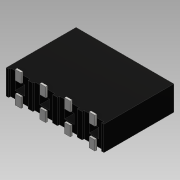
# Autodesk Inventor part: fciconnect-91601-304
Saved by Autodesk Inventor 2016 (Build 200138000, 138)
## iProperties
Created: 2016-06-08
Part Number: fciconnect-91601-304
Material: Generic
Document SubType Name: Modeling
Designer: admin
Density: 1 g/cm^3
Appearance: Default
Mass: 0.150532 g
Surface Area: 3.43025 cm^2
Volume: 0.150532 cm^3
Author: admin
Autodesk Inventor part; units mm, degrees
ref_plane "YZ Plane" through (0, 0, 0) normal (1, 0, 0) x (0, 1, 0)
ref_plane "XZ Plane" through (0, 0, 0) normal (0, 1, 0) x (-1, 0, 0)
ref_plane "XY Plane" through (0, 0, 0) normal (0, 0, 1) x (1, 0, 0)
sketch "Sketch1" plane through (0, 0, 0) normal (0, 0, 1) x (1, 0, 0)
  line L0 (-5.04, 3.6) -> (5.04, 3.6)
  line L1 (5.04, 3.6) -> (5.04, -3.6)
  line L2 (-5.04, -3.6) -> (-5.04, 3.6)
  line L3 (-2.79, -3.4) -> (-2.79, -3.6)
  line L4 (-2.79, -3.6) -> (-2.29, -3.6)
  line L5 (-2.29, -3.6) -> (-2.29, -3.4)
  line L6 (-0.25, -3.4) -> (-0.25, -3.6)
  line L7 (-0.25, -3.6) -> (0.25, -3.6)
  line L8 (0.25, -3.6) -> (0.25, -3.4)
  line L9 (2.29, -3.4) -> (2.29, -3.6)
  line L10 (2.29, -3.6) -> (2.79, -3.6)
  line L11 (2.79, -3.6) -> (2.79, -3.4)
  line L12 (-2.79, -3.4) -> (-4.79, -3.4)
  line L13 (-0.25, -3.4) -> (-2.29, -3.4)
  line L14 (4.79, -3.4) -> (2.79, -3.4)
  line L15 (2.29, -3.4) -> (0.25, -3.4)
  line L16 (0, 1.3653) -> (0, -1.7187) construction
  line L17 (-4.79, -3.4) -> (-4.79, -3.6)
  line L18 (-4.79, -3.6) -> (-5.04, -3.6)
  line L19 (4.79, -3.4) -> (4.79, -3.6)
  line L20 (4.79, -3.6) -> (5.04, -3.6)
  point P0 (0, 0)
  point P1 (0, 3.6)
  point P2 (-5.04, 0)
  point P3 (0, -3.6)
  point P4 (-2.54, -3.6)
  point P5 (-2.54, -3.6)
  point P6 (5.04, 0)
  dimension "d0" = 0.5
  dimension "d1" = 0.2
  dimension "d3" = 10.08
  dimension "d4" = 2.54
  dimension "d20" = 7
  dimension "d21" = 0.25
  constraints: 44 end point, 9 vertical, 8 collinear, 5 midpoint, 5 parallel, 5 point on line, 4 horizontal, 2 horizontal alignment, 2 vertical alignment, 1 coincident, 1 perpendicular, 1 other
  measures "d0" distance of L3.end L4.end
  measures "d1" distance of L6.start L6.end
  measures "d3" distance of L0.start L0.end
  measures "d4" distance of point (0, -3.6) point (-2.54, -3.6)
  measures "d20" distance between parallel lines of L12 L0
  measures "d21" distance of L2.start L17.end
extrude "Extrusion1" add sketch "Sketch1" along normal blind 2.54
sketch "Sketch3" plane through (-5.04, -3.4, 0) normal (0, -1, 0) x (1, 0, 0)
  line L0 (0.93, 2.87) -> (1.53, 2.87)
  line L1 (1.53, 2.87) -> (1.53, 1.87)
  line L2 (1.53, 1.87) -> (0.93, 1.87)
  line L3 (0.93, 1.87) -> (0.93, 2.87)
  line L4 (0.93, 0.67) -> (1.53, 0.67)
  line L5 (1.53, 0.67) -> (1.53, -0.33)
  line L6 (1.53, -0.33) -> (0.93, -0.33)
  line L7 (0.93, -0.33) -> (0.93, 0.67)
  line L8 (3.47, 2.87) -> (4.07, 2.87)
  line L9 (4.07, 2.87) -> (4.07, 1.87)
  line L10 (4.07, 1.87) -> (3.47, 1.87)
  line L11 (3.47, 1.87) -> (3.47, 2.87)
  line L12 (3.47, 0.67) -> (4.07, 0.67)
  line L13 (4.07, 0.67) -> (4.07, -0.33)
  line L14 (4.07, -0.33) -> (3.47, -0.33)
  line L15 (3.47, -0.33) -> (3.47, 0.67)
  line L16 (6.01, 2.87) -> (6.61, 2.87)
  line L17 (6.61, 2.87) -> (6.61, 1.87)
  line L18 (6.61, 1.87) -> (6.01, 1.87)
  line L19 (6.01, 1.87) -> (6.01, 2.87)
  line L20 (6.01, 0.67) -> (6.61, 0.67)
  line L21 (6.61, 0.67) -> (6.61, -0.33)
  line L22 (6.61, -0.33) -> (6.01, -0.33)
  line L23 (6.01, -0.33) -> (6.01, 0.67)
  line L24 (8.55, 2.87) -> (9.15, 2.87)
  line L25 (9.15, 2.87) -> (9.15, 1.87)
  line L26 (9.15, 1.87) -> (8.55, 1.87)
  line L27 (8.55, 1.87) -> (8.55, 2.87)
  line L28 (8.55, 0.67) -> (9.15, 0.67)
  line L29 (9.15, 0.67) -> (9.15, -0.33)
  line L30 (9.15, -0.33) -> (8.55, -0.33)
  line L31 (8.55, -0.33) -> (8.55, 0.67)
  line L32 (4.79, 0) -> (2.75, 0) projected
  line L33 (6.0777, 1.27) -> (8.8799, 1.27) construction
  line L34 (0, 0) -> (0, 2.54) projected
  line L35 (0, 0) -> (0, 2.54) projected
  point P0 (5.04, 0)
  point P1 (1.23, -0.33)
  point P2 (3.77, -0.33)
  point P3 (6.31, -0.33)
  point P4 (8.85, -0.33)
  point P5 (3.77, -0.33)
  point P6 (1.23, -0.33)
  point P7 (6.31, -0.33)
  point P8 (8.85, -0.33)
  point P9 (3.77, 0)
  point P10 (0, 1.27)
  dimension "d11" = 3.2
  dimension "d12" = 0.6
  dimension "d13" = 2.54
  dimension "d14" = 2.54
  dimension "d15" = 2.54
  dimension "d16" = 1
  constraints: 66 end point, 16 parallel, 12 equal length, 9 horizontal, 9 point on line, 8 perpendicular, 6 midpoint, 4 coincident, 4 collinear, 1 vertical alignment, 1 other
  measures "d11" distance between parallel lines of L6 L0
  measures "d12" distance of L0.start L0.end
  measures "d13" distance of point (3.77, -0.33) point (1.23, -0.33)
  measures "d14" distance of point (6.31, -0.33) point (3.77, -0.33)
  measures "d15" distance of point (8.85, -0.33) point (6.31, -0.33)
  measures "d16" distance of L6.end L4.start
extrude "Extrusion3" add sketch "Sketch3" along normal blind 0.2
sketch "Sketch5" plane through (-5.04, 3.6, 0) normal (0, 1, 0) x (1, 0, 0)
  line L0 (0, 0) -> (10.08, 0) projected
  line L1 (0, 0) -> (0, -2.54) projected
  line L2 (10.08, -2.54) -> (0, -2.54) projected
  line L3 (10.08, 0) -> (10.08, -2.54) projected
  line L4 (0.73, -0.77) -> (1.73, -0.77)
  line L5 (1.73, -0.77) -> (1.73, -1.77)
  line L6 (1.73, -1.77) -> (0.73, -1.77)
  line L7 (0.73, -1.77) -> (0.73, -0.77)
  line L8 (1.53, 0.33) -> (0.93, 0.33) projected
  point P0 (5.04, 0)
  point P1 (0.73, -1.27)
  point P2 (0, -1.27)
  point P3 (1.23, -0.77)
  point P4 (1.23, 0.33)
  dimension "d23" = 1
  constraints: 8 end point, 4 midpoint, 2 parallel, 2 perpendicular, 1 horizontal, 1 horizontal alignment, 1 vertical alignment
  measures "d23" distance of L5.end L6.end
extrude "Extrusion4" cut sketch "Sketch5" against normal blind 7 contours L4 L5 L6 L7
chamfer "Chamfer1" distance 0.5 angle 45 4 edges at (-3.81, 3.6, 0.77) (-3.31, 3.6, 1.27) (-4.31, 3.6, 1.27) (-3.81, 3.6, 1.77)
pattern_linear "Rectangular Pattern1" count 4 spacing 2.54 along (1, 0, 0) of "Extrusion4", "Chamfer1"
equation "\"d14\" = d13"
equation "\"d15\" = d13"
body "Solid1"
